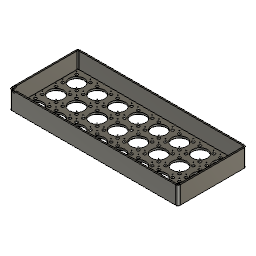
clockclock24 (Autodesk Fusion 360 design; units mm, degrees)
Autodesk Fusion 360 part; units mm, degrees
(part 1 of 2)
sketch "Sketch2" plane through (0, 0, 0) normal (0, 0, 1) x (1, 0, 0)
  circle A0 centre (0, 0) radius 16.1
  circle A1 centre (-15, 15) radius 0.95
  circle A2 centre (15, 15) radius 0.95
  circle A3 centre (-15, -15) radius 0.95
  circle A4 centre (15, -15) radius 0.95
  circle A5 centre (59.5, 15) radius 0.95
  circle A6 centre (59.5, -15) radius 0.95
  circle A7 centre (44.5, 0) radius 16.1
  circle A8 centre (29.5, 15) radius 0.95
  circle A9 centre (29.5, -15) radius 0.95
  circle A10 centre (104, 15) radius 0.95
  circle A11 centre (104, -15) radius 0.95
  circle A12 centre (89, 0) radius 16.1
  circle A13 centre (74, 15) radius 0.95
  circle A14 centre (74, -15) radius 0.95
  circle A15 centre (148.5, 15) radius 0.95
  circle A16 centre (148.5, -15) radius 0.95
  circle A17 centre (133.5, 0) radius 16.1
  circle A18 centre (118.5, 15) radius 0.95
  circle A19 centre (118.5, -15) radius 0.95
  circle A20 centre (193, 15) radius 0.95
  circle A21 centre (193, -15) radius 0.95
  circle A22 centre (178, 0) radius 16.1
  circle A23 centre (163, 15) radius 0.95
  circle A24 centre (163, -15) radius 0.95
  circle A25 centre (237.5, 15) radius 0.95
  circle A26 centre (237.5, -15) radius 0.95
  circle A27 centre (222.5, 0) radius 16.1
  circle A28 centre (207.5, 15) radius 0.95
  circle A29 centre (207.5, -15) radius 0.95
  circle A30 centre (282, 15) radius 0.95
  circle A31 centre (282, -15) radius 0.95
  circle A32 centre (267, 0) radius 16.1
  circle A33 centre (252, 15) radius 0.95
  circle A34 centre (252, -15) radius 0.95
  circle A35 centre (326.5, 15) radius 0.95
  circle A36 centre (326.5, -15) radius 0.95
  circle A37 centre (311.5, 0) radius 16.1
  circle A38 centre (296.5, 15) radius 0.95
  circle A39 centre (296.5, -15) radius 0.95
  circle A40 centre (15, 59.5) radius 0.95
  circle A41 centre (15, 29.5) radius 0.95
  circle A42 centre (0, 44.5) radius 16.1
  circle A43 centre (-15, 59.5) radius 0.95
  circle A44 centre (-15, 29.5) radius 0.95
  circle A45 centre (59.5, 59.5) radius 0.95
  circle A46 centre (59.5, 29.5) radius 0.95
  circle A47 centre (44.5, 44.5) radius 16.1
  circle A48 centre (29.5, 59.5) radius 0.95
  circle A49 centre (29.5, 29.5) radius 0.95
  circle A50 centre (104, 59.5) radius 0.95
  circle A51 centre (104, 29.5) radius 0.95
  circle A52 centre (89, 44.5) radius 16.1
  circle A53 centre (74, 59.5) radius 0.95
  circle A54 centre (74, 29.5) radius 0.95
  circle A55 centre (148.5, 59.5) radius 0.95
  circle A56 centre (148.5, 29.5) radius 0.95
  circle A57 centre (133.5, 44.5) radius 16.1
  circle A58 centre (118.5, 59.5) radius 0.95
  circle A59 centre (118.5, 29.5) radius 0.95
  circle A60 centre (193, 59.5) radius 0.95
  circle A61 centre (193, 29.5) radius 0.95
  circle A62 centre (178, 44.5) radius 16.1
  circle A63 centre (163, 59.5) radius 0.95
  circle A64 centre (163, 29.5) radius 0.95
  circle A65 centre (237.5, 59.5) radius 0.95
  circle A66 centre (237.5, 29.5) radius 0.95
  circle A67 centre (222.5, 44.5) radius 16.1
  circle A68 centre (207.5, 59.5) radius 0.95
  circle A69 centre (207.5, 29.5) radius 0.95
  circle A70 centre (282, 59.5) radius 0.95
  circle A71 centre (282, 29.5) radius 0.95
  circle A72 centre (267, 44.5) radius 16.1
  circle A73 centre (252, 59.5) radius 0.95
  circle A74 centre (252, 29.5) radius 0.95
  circle A75 centre (326.5, 59.5) radius 0.95
  circle A76 centre (326.5, 29.5) radius 0.95
  circle A77 centre (311.5, 44.5) radius 16.1
  circle A78 centre (296.5, 59.5) radius 0.95
  circle A79 centre (296.5, 29.5) radius 0.95
  circle A80 centre (15, 104) radius 0.95
  circle A81 centre (15, 74) radius 0.95
  circle A82 centre (0, 89) radius 16.1
  circle A83 centre (-15, 104) radius 0.95
  circle A84 centre (-15, 74) radius 0.95
  circle A85 centre (59.5, 104) radius 0.95
  circle A86 centre (59.5, 74) radius 0.95
  circle A87 centre (44.5, 89) radius 16.1
  circle A88 centre (29.5, 104) radius 0.95
  circle A89 centre (29.5, 74) radius 0.95
  circle A90 centre (104, 104) radius 0.95
  circle A91 centre (104, 74) radius 0.95
  circle A92 centre (89, 89) radius 16.1
  circle A93 centre (74, 104) radius 0.95
  circle A94 centre (74, 74) radius 0.95
  circle A95 centre (148.5, 104) radius 0.95
  circle A96 centre (148.5, 74) radius 0.95
  circle A97 centre (133.5, 89) radius 16.1
  circle A98 centre (118.5, 104) radius 0.95
  circle A99 centre (118.5, 74) radius 0.95
  circle A100 centre (193, 104) radius 0.95
  circle A101 centre (193, 74) radius 0.95
  circle A102 centre (178, 89) radius 16.1
  circle A103 centre (163, 104) radius 0.95
  circle A104 centre (163, 74) radius 0.95
  circle A105 centre (237.5, 104) radius 0.95
  circle A106 centre (237.5, 74) radius 0.95
  circle A107 centre (222.5, 89) radius 16.1
  circle A108 centre (207.5, 104) radius 0.95
  circle A109 centre (207.5, 74) radius 0.95
  circle A110 centre (282, 104) radius 0.95
  circle A111 centre (282, 74) radius 0.95
  circle A112 centre (267, 89) radius 16.1
  circle A113 centre (252, 104) radius 0.95
  circle A114 centre (252, 74) radius 0.95
  circle A115 centre (326.5, 104) radius 0.95
  circle A116 centre (326.5, 74) radius 0.95
  circle A117 centre (311.5, 89) radius 16.1
  circle A118 centre (296.5, 104) radius 0.95
  circle A119 centre (296.5, 74) radius 0.95
  line L0 (-22, -30) -> (333.5, -30)
  line L1 (338.5, -25) -> (338.5, 114)
  line L2 (333.5, 119) -> (-22, 119)
  line L3 (-27, 114) -> (-27, -25)
  arc A120 (338.5, 114) -> (333.5, 119) centre (333.5, 114) ccw
  arc A121 (-22, 119) -> (-27, 114) centre (-22, 114) ccw
  arc A122 (-27, -25) -> (-22, -30) centre (-22, -25) ccw
  arc A123 (333.5, -30) -> (338.5, -25) centre (333.5, -25) ccw
  point P0 (44.5, 0)
  point P1 (89, 0)
  point P2 (133.5, 0)
  point P3 (178, 0)
  point P4 (222.5, 0)
  point P5 (267, 0)
  point P6 (311.5, 0)
  point P7 (0, 44.5)
  point P8 (44.5, 44.5)
  point P9 (89, 44.5)
  point P10 (133.5, 44.5)
  point P11 (178, 44.5)
  point P12 (222.5, 44.5)
  point P13 (267, 44.5)
  point P14 (311.5, 44.5)
  point P15 (0, 89)
  point P16 (44.5, 89)
  point P17 (89, 89)
  point P18 (133.5, 89)
  point P19 (178, 89)
  point P20 (222.5, 89)
  point P21 (267, 89)
  point P22 (311.5, 89)
  point P23 (-27, -30)
  point P24 (338.5, -30)
  dimension "d3" = 32.2
  dimension "d5" = 15
  dimension "d6" = 15
  dimension "d7" = 1.9
  dimension "d10" = 30
  dimension "d11" = -30
  dimension "d14" = 311.5
  dimension "d15" = 89
  dimension "d17" = 27
  dimension "d18" = 27
  dimension "d19" = 30
  dimension "d20" = 30
  dimension "d22" = 365.5
  dimension "d41" = 5
  constraint coincident A0.centre origin
  constraint horizontal L0
  constraint vertical L1
  constraint horizontal L2
  constraint vertical L3
  constraint tangent L1 A120
  constraint tangent L2 A120
  constraint tangent L2 A121
  constraint tangent L3 A121
  constraint equal A120 A121
  constraint coincident P23 L0
  constraint coincident P23 L3
  constraint tangent L0 A122
  constraint tangent L3 A122
  constraint equal A120 A122
  constraint coincident P24 L0
  constraint coincident P24 L1
  constraint tangent L0 A123
  constraint tangent L1 A123
  constraint equal A120 A123
  measures "d3" diameter of A0
  measures "d5" horizontal distance of A0.centre A1.centre
  measures "d6" vertical distance of A0.centre A1.centre
  measures "d7" diameter of A1
  measures "d17" distance of P7 L3
  measures "d18" distance of P14 L1
  measures "d19" distance of P22 L2
  measures "d20" distance of P6 L0
  measures "d22" distance of P23 P24
  measures "d41" radius of A120
extrude "Extrude2" add sketch "Sketch2" along normal blind 5 contours A1 | A2 | A3 | A4 | A5 | A6 | A8 | A9 | A10 | A11 | A13 | A14 | A15 | A16 | A18 | A19 | A20 | A21 | A23 | A24 | A25 | A26 | A28 | A29 | A30 | A31 | A33 | A34 | A35 | A36 | A38 | A39 | A40 | A41 | A43 | A44 | A45 | A46 | A48 | A49 | A50 | A51 | A53 | A54 | A55 | A56 | A58 | A59 | A60 | A61 | A63 | A64 | A65 | A66 | A68 | A69 | A70 | A71 | A73 | A74 | A75 | A76 | A78 | A79 | A80 | A81 | A83 | A84 | A85 | A86 | A88 | A89 | A90 | A91 | A93 | A94 | A95 | A96 | A98 | A99 | A100 | A101 | A103 | A104 | A105 | A106 | A108 | A109 | A110 | A111 | A113 | A114 | A115 | A116 | A118 | A119 | L0 L1 L2 L3 A120 A121 A122 A123 makes body 1
extrude "Extrude3" add sketch "Sketch2" along normal blind 11 contours A1 | A2 | A3 | A4 | A5 | A6 | A8 | A9 | A10 | A11 | A13 | A14 | A15 | A16 | A18 | A19 | A20 | A21 | A23 | A24 | A25 | A26 | A28 | A29 | A30 | A31 | A33 | A34 | A35 | A36 | A38 | A39 | A40 | A41 | A43 | A44 | A45 | A46 | A48 | A49 | A50 | A51 | A53 | A54 | A55 | A56 | A58 | A59 | A60 | A61 | A63 | A64 | A65 | A66 | A68 | A69 | A70 | A71 | A73 | A74 | A75 | A76 | A78 | A79 | A80 | A81 | A83 | A84 | A85 | A86 | A88 | A89 | A90 | A91 | A93 | A94 | A95 | A96 | A98 | A99 | A100 | A101 | A103 | A104 | A105 | A106 | A108 | A109 | A110 | A111 | A113 | A114 | A115 | A116 | A118 | A119 bodies 1
extrude "Extrude5" add sketch "Sketch2" along normal blind 40 thin wall 3 on the right open curves L3 A122 L0 A123 L1 A120 L2 A121 bodies 1
fillet "Fillet1" radius 2 96 edges at (-15.8857, -14.6565, 5) (14.1143, -14.6565, 5) (28.6143, -14.6565, 5) (58.6143, -14.6565, 5) (58.6143, 15.3435, 5) (28.6143, 15.3435, 5) (14.1143, 15.3435, 5) (-15.8857, 15.3435, 5) (-15.8857, 29.8435, 5) (-15.8857, 59.8435, 5) (-15.8857, 74.3435, 5) (-15.8857, 104.3435, 5) (14.1143, 104.3435, 5) (28.6143, 104.3435, 5) (58.6143, 104.3435, 5) (73.1143, 104.3435, 5) (73.1143, 74.3435, 5) (58.6143, 74.3435, 5) (28.6143, 59.8435, 5) (14.1143, 59.8435, 5) (14.1143, 74.3435, 5) (28.6143, 74.3435, 5) (58.6143, 59.8435, 5) (73.1143, 59.8435, 5) (58.6143, 29.8435, 5) (73.1143, 29.8435, 5) (28.6143, 29.8435, 5) (14.1143, 29.8435, 5) (73.1143, 15.3435, 5) (73.1143, -14.6565, 5) (103.1143, -14.6565, 5) (103.1143, 15.3435, 5) (103.1143, 29.8435, 5) (103.1143, 59.8435, 5) (103.1143, 74.3435, 5) (103.1143, 104.3435, 5) (117.6143, 104.3435, 5) (117.6143, 74.3435, 5) (117.6143, 59.8435, 5) (117.6143, 29.8435, 5) (117.6143, 15.3435, 5) (117.6143, -14.6565, 5) (147.6143, -14.6565, 5) (147.6143, 15.3435, 5) (147.6143, 29.8435, 5) (147.6143, 59.8435, 5) (147.6143, 74.3435, 5) (147.6143, 104.3435, 5) (162.1143, 104.3435, 5) (162.1143, 74.3435, 5) (162.1143, 59.8435, 5) (162.1143, 29.8435, 5) (162.1143, 15.3435, 5) (162.1143, -14.6565, 5) (192.1143, -14.6565, 5) (192.1143, 15.3435, 5) (192.1143, 29.8435, 5) (192.1143, 59.8435, 5) (192.1143, 74.3435, 5) (192.1143, 104.3435, 5) (206.6143, 104.3435, 5) (236.6143, 104.3435, 5) (251.1143, 104.3435, 5) (281.1143, 104.3435, 5) (295.6143, 104.3435, 5) (206.6143, 74.3435, 5) (236.6143, 74.3435, 5) (251.1143, 74.3435, 5) (281.1143, 74.3435, 5) (295.6143, 74.3435, 5) (295.6143, 59.8435, 5) (281.1143, 59.8435, 5) (251.1143, 59.8435, 5) (236.6143, 59.8435, 5) (206.6143, 59.8435, 5) (206.6143, 29.8435, 5) (236.6143, 29.8435, 5) (251.1143, 29.8435, 5) (281.1143, 29.8435, 5) (295.6143, 29.8435, 5) (325.6143, 29.8435, 5) (325.6143, 15.3435, 5) (295.6143, 15.3435, 5) (281.1143, 15.3435, 5) (251.1143, 15.3435, 5) (325.6143, -14.6565, 5) (295.6143, -14.6565, 5) (281.1143, -14.6565, 5) (251.1143, -14.6565, 5) (236.6143, -14.6565, 5) (236.6143, 15.3435, 5) (206.6143, 15.3435, 5) (206.6143, -14.6565, 5) (325.6143, 104.3435, 5) (325.6143, 74.3435, 5) (325.6143, 59.8435, 5) on bodies 1
sketch "DXF_PCB3_2026-08-19_AutoCAD2007" plane through (0, 0, 0) normal (0, 0, 1) x (1, 0, 0)
  line L0 (-17, -130.4333) -> (-17, -0.301)
  arc A0 (-12, -135.4333) -> (-17, -130.4333) centre (-11.9982, -130.4314) cw
  arc A1 (17, -130.4333) -> (12, -135.4333) centre (11.9982, -130.4314) cw
  line L1 (12, -135.4333) -> (-12, -135.4333)
  arc A2 (12, 4.699) -> (17, -0.301) centre (11.9982, -0.3028) cw
  line L2 (17, -0.301) -> (17, -130.4333)
  line L3 (-12, 4.699) -> (12, 4.699)
  arc A3 (-17, -0.301) -> (-12, 4.699) centre (-11.9982, -0.3028) cw
  arc A4 (-11.722, 1) -> (-15.278, 1) centre (-13.5, 1) ccw
  arc A5 (-15.278, 1) -> (-11.722, 1) centre (-13.5, 1) ccw
  arc A6 (11.722, 1) -> (15.278, 1) centre (13.5, 1) ccw
  arc A7 (15.278, 1) -> (11.722, 1) centre (13.5, 1) ccw
  arc A8 (-11.849, -131.0003) -> (-15.405, -131.0003) centre (-13.627, -131.0003) ccw
  arc A9 (-15.405, -131.0003) -> (-11.849, -131.0003) centre (-13.627, -131.0003) ccw
  arc A10 (11.595, -131.0003) -> (15.151, -131.0003) centre (13.373, -131.0003) ccw
  arc A11 (15.151, -131.0003) -> (11.595, -131.0003) centre (13.373, -131.0003) ccw
  arc A12 (0.4999, -121.4122) -> (1.9999, -121.4122) centre (1.2499, -121.4122) ccw
  arc A13 (1.9999, -121.4122) -> (0.4999, -121.4122) centre (1.2499, -121.4122) ccw
  arc A14 (1.9999, -121.4122) -> (0.4999, -121.4122) centre (1.2499, -121.4122) ccw
  arc A15 (0.4999, -121.4122) -> (1.9999, -121.4122) centre (1.2499, -121.4122) ccw
  arc A16 (0.4999, -121.4122) -> (1.9999, -121.4122) centre (1.2499, -121.4122) ccw
  arc A17 (1.9999, -121.4122) -> (0.4999, -121.4122) centre (1.2499, -121.4122) ccw
  arc A18 (-1.9999, -121.4122) -> (-0.4999, -121.4122) centre (-1.2499, -121.4122) ccw
  arc A19 (-0.4999, -121.4122) -> (-1.9999, -121.4122) centre (-1.2499, -121.4122) ccw
  arc A20 (-1.9999, -121.4122) -> (-0.4999, -121.4122) centre (-1.2499, -121.4122) ccw
  arc A21 (-0.4999, -121.4122) -> (-1.9999, -121.4122) centre (-1.2499, -121.4122) ccw
  arc A22 (-1.9999, -121.4122) -> (-0.4999, -121.4122) centre (-1.2499, -121.4122) ccw
  arc A23 (-0.4999, -121.4122) -> (-1.9999, -121.4122) centre (-1.2499, -121.4122) ccw
  arc A24 (0.47, -96.0122) -> (2.07, -96.0122) centre (1.27, -96.0122) ccw
  arc A25 (2.07, -96.0122) -> (0.47, -96.0122) centre (1.27, -96.0122) ccw
  arc A26 (0.47, -96.0122) -> (2.07, -96.0122) centre (1.27, -96.0122) ccw
  arc A27 (2.07, -96.0122) -> (0.47, -96.0122) centre (1.27, -96.0122) ccw
  arc A28 (2.07, -96.0122) -> (0.47, -96.0122) centre (1.27, -96.0122) ccw
  arc A29 (0.47, -96.0122) -> (2.07, -96.0122) centre (1.27, -96.0122) ccw
  arc A30 (-2.07, -96.0122) -> (-0.47, -96.0122) centre (-1.27, -96.0122) ccw
  arc A31 (-0.47, -96.0122) -> (-2.07, -96.0122) centre (-1.27, -96.0122) ccw
  arc A32 (-2.07, -96.0122) -> (-0.47, -96.0122) centre (-1.27, -96.0122) ccw
  arc A33 (-0.47, -96.0122) -> (-2.07, -96.0122) centre (-1.27, -96.0122) ccw
  arc A34 (-2.07, -96.0122) -> (-0.47, -96.0122) centre (-1.27, -96.0122) ccw
  arc A35 (-0.47, -96.0122) -> (-2.07, -96.0122) centre (-1.27, -96.0122) ccw
  line L4 (-7.1, -63.6671) -> (-7.1, -63.6671)
  arc A36 (-7.1, -63.6671) -> (-8.9, -63.6671) centre (-8, -63.6671) ccw
  arc A37 (-8.9, -63.6671) -> (-7.1, -63.6671) centre (-8, -63.6671) ccw
  arc A38 (-8.9, -63.6671) -> (-7.1, -63.6671) centre (-8, -63.6671) ccw
  arc A39 (-7.1, -63.6671) -> (-8.9, -63.6671) centre (-8, -63.6671) ccw
  line L5 (-7.1, -63.6671) -> (-7.1, -63.6671)
  line L6 (-7.1, -63.6671) -> (-7.1, -63.6671)
  arc A40 (-7.1, -63.6671) -> (-8.9, -63.6671) centre (-8, -63.6671) ccw
  arc A41 (-8.9, -63.6671) -> (-7.1, -63.6671) centre (-8, -63.6671) ccw
  arc A42 (-7.1, -66.167) -> (-8.9, -66.167) centre (-8, -66.167) ccw
  arc A43 (-8.9, -66.167) -> (-7.1, -66.167) centre (-8, -66.167) ccw
  arc A44 (-7.1, -66.167) -> (-8.9, -66.167) centre (-8, -66.167) ccw
  arc A45 (-8.9, -66.167) -> (-7.1, -66.167) centre (-8, -66.167) ccw
  arc A46 (-7.1, -66.167) -> (-8.9, -66.167) centre (-8, -66.167) ccw
  arc A47 (-8.9, -66.167) -> (-7.1, -66.167) centre (-8, -66.167) ccw
  arc A48 (-7.1, -68.6671) -> (-8.9, -68.6671) centre (-8, -68.6671) ccw
  arc A49 (-8.9, -68.6671) -> (-7.1, -68.6671) centre (-8, -68.6671) ccw
  line L7 (-7.1, -68.6671) -> (-7.1, -68.6671)
  line L8 (-7.1, -68.6671) -> (-7.1, -68.6671)
  arc A50 (-7.1, -68.6671) -> (-8.9, -68.6671) centre (-8, -68.6671) ccw
  arc A51 (-8.9, -68.6671) -> (-7.1, -68.6671) centre (-8, -68.6671) ccw
  arc A52 (-7.1, -68.6671) -> (-8.9, -68.6671) centre (-8, -68.6671) ccw
  line L9 (-7.1, -68.6671) -> (-7.1, -68.6671)
  arc A53 (-8.9, -68.6671) -> (-7.1, -68.6671) centre (-8, -68.6671) ccw
  arc A54 (8.9, -68.6671) -> (7.1, -68.6671) centre (8, -68.6671) ccw
  arc A55 (7.1, -68.6671) -> (8.9, -68.6671) centre (8, -68.6671) ccw
  arc A56 (7.1, -68.6671) -> (8.9, -68.6671) centre (8, -68.6671) ccw
  arc A57 (8.9, -68.6671) -> (7.1, -68.6671) centre (8, -68.6671) ccw
  arc A58 (8.9, -68.6671) -> (7.1, -68.6671) centre (8, -68.6671) ccw
  arc A59 (7.1, -68.6671) -> (8.9, -68.6671) centre (8, -68.6671) ccw
  arc A60 (8.9, -66.1673) -> (7.1, -66.1673) centre (8, -66.1673) ccw
  arc A61 (7.1, -66.1673) -> (8.9, -66.1673) centre (8, -66.1673) ccw
  arc A62 (7.1, -66.1673) -> (8.9, -66.1673) centre (8, -66.1673) ccw
  arc A63 (8.9, -66.1673) -> (7.1, -66.1673) centre (8, -66.1673) ccw
  arc A64 (8.9, -66.1673) -> (7.1, -66.1673) centre (8, -66.1673) ccw
  arc A65 (7.1, -66.1673) -> (8.9, -66.1673) centre (8, -66.1673) ccw
  arc A66 (7.1, -63.6671) -> (8.9, -63.6671) centre (8, -63.6671) ccw
  arc A67 (8.9, -63.6671) -> (7.1, -63.6671) centre (8, -63.6671) ccw
  arc A68 (7.1, -63.6671) -> (8.9, -63.6671) centre (8, -63.6671) ccw
  arc A69 (8.9, -63.6671) -> (7.1, -63.6671) centre (8, -63.6671) ccw
  arc A70 (7.1, -63.6671) -> (8.9, -63.6671) centre (8, -63.6671) ccw
  arc A71 (8.9, -63.6671) -> (7.1, -63.6671) centre (8, -63.6671) ccw
  arc A72 (7.112, -12.573) -> (8.636, -12.573) centre (7.874, -12.573) ccw
  arc A73 (8.636, -12.573) -> (7.112, -12.573) centre (7.874, -12.573) ccw
  arc A74 (8.636, -12.573) -> (7.112, -12.573) centre (7.874, -12.573) ccw
  arc A75 (7.112, -12.573) -> (8.636, -12.573) centre (7.874, -12.573) ccw
  arc A76 (8.636, -12.573) -> (7.112, -12.573) centre (7.874, -12.573) ccw
  arc A77 (7.112, -12.573) -> (8.636, -12.573) centre (7.874, -12.573) ccw
  arc A78 (4.572, -12.573) -> (6.096, -12.573) centre (5.334, -12.573) ccw
  arc A79 (6.096, -12.573) -> (4.572, -12.573) centre (5.334, -12.573) ccw
  arc A80 (6.096, -12.573) -> (4.572, -12.573) centre (5.334, -12.573) ccw
  arc A81 (4.572, -12.573) -> (6.096, -12.573) centre (5.334, -12.573) ccw
  arc A82 (6.096, -12.573) -> (4.572, -12.573) centre (5.334, -12.573) ccw
  arc A83 (4.572, -12.573) -> (6.096, -12.573) centre (5.334, -12.573) ccw
  arc A84 (2.032, -12.573) -> (3.556, -12.573) centre (2.794, -12.573) ccw
  arc A85 (3.556, -12.573) -> (2.032, -12.573) centre (2.794, -12.573) ccw
  arc A86 (3.556, -12.573) -> (2.032, -12.573) centre (2.794, -12.573) ccw
  arc A87 (2.032, -12.573) -> (3.556, -12.573) centre (2.794, -12.573) ccw
  arc A88 (3.556, -12.573) -> (2.032, -12.573) centre (2.794, -12.573) ccw
  arc A89 (2.032, -12.573) -> (3.556, -12.573) centre (2.794, -12.573) ccw
  arc A90 (-0.508, -12.573) -> (1.016, -12.573) centre (0.254, -12.573) ccw
  arc A91 (1.016, -12.573) -> (-0.508, -12.573) centre (0.254, -12.573) ccw
  arc A92 (1.016, -12.573) -> (-0.508, -12.573) centre (0.254, -12.573) ccw
  arc A93 (-0.508, -12.573) -> (1.016, -12.573) centre (0.254, -12.573) ccw
  arc A94 (1.016, -12.573) -> (-0.508, -12.573) centre (0.254, -12.573) ccw
  arc A95 (-0.508, -12.573) -> (1.016, -12.573) centre (0.254, -12.573) ccw
  arc A96 (-1.524, -12.573) -> (-3.048, -12.573) centre (-2.286, -12.573) ccw
  arc A97 (-3.048, -12.573) -> (-1.524, -12.573) centre (-2.286, -12.573) ccw
  arc A98 (-3.048, -12.573) -> (-1.524, -12.573) centre (-2.286, -12.573) ccw
  arc A99 (-1.524, -12.573) -> (-3.048, -12.573) centre (-2.286, -12.573) ccw
  arc A100 (-3.048, -12.573) -> (-1.524, -12.573) centre (-2.286, -12.573) ccw
  arc A101 (-1.524, -12.573) -> (-3.048, -12.573) centre (-2.286, -12.573) ccw
  arc A102 (-5.588, -12.573) -> (-4.064, -12.573) centre (-4.826, -12.573) ccw
  arc A103 (-4.064, -12.573) -> (-5.588, -12.573) centre (-4.826, -12.573) ccw
  arc A104 (-4.064, -12.573) -> (-5.588, -12.573) centre (-4.826, -12.573) ccw
  arc A105 (-5.588, -12.573) -> (-4.064, -12.573) centre (-4.826, -12.573) ccw
  arc A106 (-4.064, -12.573) -> (-5.588, -12.573) centre (-4.826, -12.573) ccw
  arc A107 (-5.588, -12.573) -> (-4.064, -12.573) centre (-4.826, -12.573) ccw
  arc A108 (-6.604, -12.573) -> (-8.128, -12.573) centre (-7.366, -12.573) ccw
  arc A109 (-8.128, -12.573) -> (-6.604, -12.573) centre (-7.366, -12.573) ccw
  arc A110 (-6.604, -12.573) -> (-8.128, -12.573) centre (-7.366, -12.573) ccw
  arc A111 (-8.128, -12.573) -> (-6.604, -12.573) centre (-7.366, -12.573) ccw
  arc A112 (-6.604, -12.573) -> (-8.128, -12.573) centre (-7.366, -12.573) ccw
  arc A113 (-8.128, -12.573) -> (-6.604, -12.573) centre (-7.366, -12.573) ccw
  arc A114 (-8.128, -27.8131) -> (-6.604, -27.8131) centre (-7.366, -27.8131) ccw
  arc A115 (-6.604, -27.8131) -> (-8.128, -27.8131) centre (-7.366, -27.8131) ccw
  arc A116 (-6.604, -27.8131) -> (-8.128, -27.8131) centre (-7.366, -27.8131) ccw
  arc A117 (-8.128, -27.8131) -> (-6.604, -27.8131) centre (-7.366, -27.8131) ccw
  arc A118 (-6.604, -27.8131) -> (-8.128, -27.8131) centre (-7.366, -27.8131) ccw
  arc A119 (-8.128, -27.8131) -> (-6.604, -27.8131) centre (-7.366, -27.8131) ccw
  arc A120 (-5.588, -27.8131) -> (-4.064, -27.8131) centre (-4.826, -27.8131) ccw
  arc A121 (-4.064, -27.8131) -> (-5.588, -27.8131) centre (-4.826, -27.8131) ccw
  arc A122 (-4.064, -27.8131) -> (-5.588, -27.8131) centre (-4.826, -27.8131) ccw
  arc A123 (-5.588, -27.8131) -> (-4.064, -27.8131) centre (-4.826, -27.8131) ccw
  arc A124 (-5.588, -27.8131) -> (-4.064, -27.8131) centre (-4.826, -27.8131) ccw
  arc A125 (-4.064, -27.8131) -> (-5.588, -27.8131) centre (-4.826, -27.8131) ccw
  arc A126 (-3.048, -27.8131) -> (-1.524, -27.8131) centre (-2.286, -27.8131) ccw
  arc A127 (-1.524, -27.8131) -> (-3.048, -27.8131) centre (-2.286, -27.8131) ccw
  arc A128 (-3.048, -27.8131) -> (-1.524, -27.8131) centre (-2.286, -27.8131) ccw
  arc A129 (-1.524, -27.8131) -> (-3.048, -27.8131) centre (-2.286, -27.8131) ccw
  arc A130 (-3.048, -27.8131) -> (-1.524, -27.8131) centre (-2.286, -27.8131) ccw
  arc A131 (-1.524, -27.8131) -> (-3.048, -27.8131) centre (-2.286, -27.8131) ccw
  arc A132 (-0.508, -27.8131) -> (1.016, -27.8131) centre (0.254, -27.8131) ccw
  arc A133 (1.016, -27.8131) -> (-0.508, -27.8131) centre (0.254, -27.8131) ccw
  arc A134 (-0.508, -27.8131) -> (1.016, -27.8131) centre (0.254, -27.8131) ccw
  arc A135 (1.016, -27.8131) -> (-0.508, -27.8131) centre (0.254, -27.8131) ccw
  arc A136 (1.016, -27.8131) -> (-0.508, -27.8131) centre (0.254, -27.8131) ccw
  arc A137 (-0.508, -27.8131) -> (1.016, -27.8131) centre (0.254, -27.8131) ccw
  arc A138 (2.032, -27.8131) -> (3.556, -27.8131) centre (2.794, -27.8131) ccw
  arc A139 (3.556, -27.8131) -> (2.032, -27.8131) centre (2.794, -27.8131) ccw
  arc A140 (3.556, -27.8131) -> (2.032, -27.8131) centre (2.794, -27.8131) ccw
  arc A141 (2.032, -27.8131) -> (3.556, -27.8131) centre (2.794, -27.8131) ccw
  arc A142 (3.556, -27.8131) -> (2.032, -27.8131) centre (2.794, -27.8131) ccw
  arc A143 (2.032, -27.8131) -> (3.556, -27.8131) centre (2.794, -27.8131) ccw
  arc A144 (4.572, -27.8131) -> (6.096, -27.8131) centre (5.334, -27.8131) ccw
  arc A145 (6.096, -27.8131) -> (4.572, -27.8131) centre (5.334, -27.8131) ccw
  arc A146 (6.096, -27.8131) -> (4.572, -27.8131) centre (5.334, -27.8131) ccw
  arc A147 (4.572, -27.8131) -> (6.096, -27.8131) centre (5.334, -27.8131) ccw
  arc A148 (6.096, -27.8131) -> (4.572, -27.8131) centre (5.334, -27.8131) ccw
  arc A149 (4.572, -27.8131) -> (6.096, -27.8131) centre (5.334, -27.8131) ccw
  arc A150 (7.112, -27.8131) -> (8.636, -27.8131) centre (7.874, -27.8131) ccw
  arc A151 (8.636, -27.8131) -> (7.112, -27.8131) centre (7.874, -27.8131) ccw
  arc A152 (8.636, -27.8131) -> (7.112, -27.8131) centre (7.874, -27.8131) ccw
  arc A153 (7.112, -27.8131) -> (8.636, -27.8131) centre (7.874, -27.8131) ccw
  arc A154 (7.112, -27.8131) -> (8.636, -27.8131) centre (7.874, -27.8131) ccw
  arc A155 (8.636, -27.8131) -> (7.112, -27.8131) centre (7.874, -27.8131) ccw
  arc A156 (-8.0404, -0.0001) -> (-9.7404, -0.0001) centre (-8.8904, -0.0001) ccw
  arc A157 (-9.7404, -0.0001) -> (-8.0404, -0.0001) centre (-8.8904, -0.0001) ccw
  arc A158 (-8.0404, -0.0001) -> (-9.7404, -0.0001) centre (-8.8904, -0.0001) ccw
  arc A159 (-9.7404, -0.0001) -> (-8.0404, -0.0001) centre (-8.8904, -0.0001) ccw
  arc A160 (-8.0404, -0.0001) -> (-9.7404, -0.0001) centre (-8.8904, -0.0001) ccw
  arc A161 (-9.7404, -0.0001) -> (-8.0404, -0.0001) centre (-8.8904, -0.0001) ccw
  arc A162 (-5.5004, -0.0001) -> (-7.2004, -0.0001) centre (-6.3504, -0.0001) ccw
  arc A163 (-7.2004, -0.0001) -> (-5.5004, -0.0001) centre (-6.3504, -0.0001) ccw
  arc A164 (-7.2004, -0.0001) -> (-5.5004, -0.0001) centre (-6.3504, -0.0001) ccw
  arc A165 (-5.5004, -0.0001) -> (-7.2004, -0.0001) centre (-6.3504, -0.0001) ccw
  arc A166 (-5.5004, -0.0001) -> (-7.2004, -0.0001) centre (-6.3504, -0.0001) ccw
  arc A167 (-7.2004, -0.0001) -> (-5.5004, -0.0001) centre (-6.3504, -0.0001) ccw
  arc A168 (-2.9604, -0.0001) -> (-4.6604, -0.0001) centre (-3.8104, -0.0001) ccw
  arc A169 (-4.6604, -0.0001) -> (-2.9604, -0.0001) centre (-3.8104, -0.0001) ccw
  arc A170 (-4.6604, -0.0001) -> (-2.9604, -0.0001) centre (-3.8104, -0.0001) ccw
  arc A171 (-2.9604, -0.0001) -> (-4.6604, -0.0001) centre (-3.8104, -0.0001) ccw
  arc A172 (-4.6604, -0.0001) -> (-2.9604, -0.0001) centre (-3.8104, -0.0001) ccw
  arc A173 (-2.9604, -0.0001) -> (-4.6604, -0.0001) centre (-3.8104, -0.0001) ccw
  arc A174 (-0.4204, -0.0001) -> (-2.1204, -0.0001) centre (-1.2704, -0.0001) ccw
  arc A175 (-2.1204, -0.0001) -> (-0.4204, -0.0001) centre (-1.2704, -0.0001) ccw
  arc A176 (-2.1204, -0.0001) -> (-0.4204, -0.0001) centre (-1.2704, -0.0001) ccw
  arc A177 (-0.4204, -0.0001) -> (-2.1204, -0.0001) centre (-1.2704, -0.0001) ccw
  arc A178 (-0.4204, -0.0001) -> (-2.1204, -0.0001) centre (-1.2704, -0.0001) ccw
  arc A179 (-2.1204, -0.0001) -> (-0.4204, -0.0001) centre (-1.2704, -0.0001) ccw
  arc A180 (0.4196, -0.0001) -> (2.1196, -0.0001) centre (1.2696, -0.0001) ccw
  arc A181 (2.1196, -0.0001) -> (0.4196, -0.0001) centre (1.2696, -0.0001) ccw
  arc A182 (2.1196, -0.0001) -> (0.4196, -0.0001) centre (1.2696, -0.0001) ccw
  arc A183 (0.4196, -0.0001) -> (2.1196, -0.0001) centre (1.2696, -0.0001) ccw
  arc A184 (0.4196, -0.0001) -> (2.1196, -0.0001) centre (1.2696, -0.0001) ccw
  arc A185 (2.1196, -0.0001) -> (0.4196, -0.0001) centre (1.2696, -0.0001) ccw
  arc A186 (2.9596, -0.0001) -> (4.6596, -0.0001) centre (3.8096, -0.0001) ccw
  arc A187 (4.6596, -0.0001) -> (2.9596, -0.0001) centre (3.8096, -0.0001) ccw
  arc A188 (2.9596, -0.0001) -> (4.6596, -0.0001) centre (3.8096, -0.0001) ccw
  arc A189 (4.6596, -0.0001) -> (2.9596, -0.0001) centre (3.8096, -0.0001) ccw
  arc A190 (2.9596, -0.0001) -> (4.6596, -0.0001) centre (3.8096, -0.0001) ccw
  arc A191 (4.6596, -0.0001) -> (2.9596, -0.0001) centre (3.8096, -0.0001) ccw
  arc A192 (5.4996, -0.0001) -> (7.1996, -0.0001) centre (6.3496, -0.0001) ccw
  arc A193 (7.1996, -0.0001) -> (5.4996, -0.0001) centre (6.3496, -0.0001) ccw
  arc A194 (5.4996, -0.0001) -> (7.1996, -0.0001) centre (6.3496, -0.0001) ccw
  arc A195 (7.1996, -0.0001) -> (5.4996, -0.0001) centre (6.3496, -0.0001) ccw
  arc A196 (7.1996, -0.0001) -> (5.4996, -0.0001) centre (6.3496, -0.0001) ccw
  arc A197 (5.4996, -0.0001) -> (7.1996, -0.0001) centre (6.3496, -0.0001) ccw
  line L10 (9.677, -0.8501) -> (8.1022, -0.8501)
  line L11 (9.677, 0.8499) -> (9.677, -0.8501)
  line L12 (8.1022, 0.8499) -> (9.677, 0.8499)
  line L13 (8.1022, -0.8501) -> (8.1022, 0.8499)
  line L14 (8.1022, -0.8501) -> (8.1022, 0.8499)
  line L15 (8.1022, 0.8499) -> (9.677, 0.8499)
  line L16 (9.677, 0.8499) -> (9.677, -0.8501)
  line L17 (9.677, -0.8501) -> (8.1022, -0.8501)
  line L18 (8.1022, -0.8501) -> (8.1022, 0.8499)
  line L19 (8.1022, 0.8499) -> (9.677, 0.8499)
  line L20 (9.677, 0.8499) -> (9.677, -0.8501)
  line L21 (9.677, -0.8501) -> (8.1022, -0.8501)
  line L22 (2.151, -128.5243) -> (2.151, -128.5243)
  arc A198 (0.351, -128.5243) -> (2.151, -128.5243) centre (1.251, -128.5243) ccw
  arc A199 (2.151, -128.5243) -> (0.351, -128.5243) centre (1.251, -128.5243) ccw
  arc A200 (0.351, -128.5243) -> (2.151, -128.5243) centre (1.251, -128.5243) ccw
  line L23 (2.151, -128.5243) -> (2.151, -128.5243)
  arc A201 (2.151, -128.5243) -> (0.351, -128.5243) centre (1.251, -128.5243) ccw
  line L24 (2.151, -128.5243) -> (2.151, -128.5243)
  arc A202 (2.151, -128.5243) -> (0.351, -128.5243) centre (1.251, -128.5243) ccw
  arc A203 (0.351, -128.5243) -> (2.151, -128.5243) centre (1.251, -128.5243) ccw
  arc A204 (-2.151, -128.5243) -> (-0.351, -128.5243) centre (-1.251, -128.5243) ccw
  arc A205 (-0.351, -128.5243) -> (-2.151, -128.5243) centre (-1.251, -128.5243) ccw
  line L25 (-0.351, -128.5243) -> (-0.351, -128.5243)
  arc A206 (-2.151, -128.5243) -> (-0.351, -128.5243) centre (-1.251, -128.5243) ccw
  arc A207 (-0.351, -128.5243) -> (-2.151, -128.5243) centre (-1.251, -128.5243) ccw
  line L26 (-0.351, -128.5243) -> (-0.351, -128.5243)
  arc A208 (-2.151, -128.5243) -> (-0.351, -128.5243) centre (-1.251, -128.5243) ccw
  arc A209 (-0.351, -128.5243) -> (-2.151, -128.5243) centre (-1.251, -128.5243) ccw
  line L27 (-0.351, -128.5243) -> (-0.351, -128.5243)
  arc A210 (-8.382, -102.1082) -> (-10.16, -102.1082) centre (-9.271, -102.1082) ccw
  arc A211 (-10.16, -102.1082) -> (-8.382, -102.1082) centre (-9.271, -102.1082) ccw
  arc A212 (-8.382, -102.1082) -> (-10.16, -102.1082) centre (-9.271, -102.1082) ccw
  arc A213 (-10.16, -102.1082) -> (-8.382, -102.1082) centre (-9.271, -102.1082) ccw
  arc A214 (-8.382, -102.1082) -> (-10.16, -102.1082) centre (-9.271, -102.1082) ccw
  arc A215 (-10.16, -102.1082) -> (-8.382, -102.1082) centre (-9.271, -102.1082) ccw
  arc A216 (-8.382, -104.6482) -> (-10.16, -104.6482) centre (-9.271, -104.6482) ccw
  arc A217 (-10.16, -104.6482) -> (-8.382, -104.6482) centre (-9.271, -104.6482) ccw
  arc A218 (-10.16, -104.6482) -> (-8.382, -104.6482) centre (-9.271, -104.6482) ccw
  arc A219 (-8.382, -104.6482) -> (-10.16, -104.6482) centre (-9.271, -104.6482) ccw
  arc A220 (-8.382, -104.6482) -> (-10.16, -104.6482) centre (-9.271, -104.6482) ccw
  arc A221 (-10.16, -104.6482) -> (-8.382, -104.6482) centre (-9.271, -104.6482) ccw
  arc A222 (-8.382, -112.7762) -> (-10.16, -112.7762) centre (-9.271, -112.7762) ccw
  arc A223 (-10.16, -112.7762) -> (-8.382, -112.7762) centre (-9.271, -112.7762) ccw
  arc A224 (-10.16, -112.7762) -> (-8.382, -112.7762) centre (-9.271, -112.7762) ccw
  arc A225 (-8.382, -112.7762) -> (-10.16, -112.7762) centre (-9.271, -112.7762) ccw
  arc A226 (-10.16, -112.7762) -> (-8.382, -112.7762) centre (-9.271, -112.7762) ccw
  arc A227 (-8.382, -112.7762) -> (-10.16, -112.7762) centre (-9.271, -112.7762) ccw
  arc A228 (-10.16, -115.3162) -> (-8.382, -115.3162) centre (-9.271, -115.3162) ccw
  arc A229 (-8.382, -115.3162) -> (-10.16, -115.3162) centre (-9.271, -115.3162) ccw
  arc A230 (-8.382, -115.3162) -> (-10.16, -115.3162) centre (-9.271, -115.3162) ccw
  arc A231 (-10.16, -115.3162) -> (-8.382, -115.3162) centre (-9.271, -115.3162) ccw
  arc A232 (-10.16, -115.3162) -> (-8.382, -115.3162) centre (-9.271, -115.3162) ccw
  arc A233 (-8.382, -115.3162) -> (-10.16, -115.3162) centre (-9.271, -115.3162) ccw
  arc A234 (10.16, -102.1082) -> (8.382, -102.1082) centre (9.271, -102.1082) ccw
  arc A235 (8.382, -102.1082) -> (10.16, -102.1082) centre (9.271, -102.1082) ccw
  arc A236 (10.16, -102.1082) -> (8.382, -102.1082) centre (9.271, -102.1082) ccw
  arc A237 (8.382, -102.1082) -> (10.16, -102.1082) centre (9.271, -102.1082) ccw
  arc A238 (8.382, -102.1082) -> (10.16, -102.1082) centre (9.271, -102.1082) ccw
  arc A239 (10.16, -102.1082) -> (8.382, -102.1082) centre (9.271, -102.1082) ccw
  arc A240 (8.382, -104.6482) -> (10.16, -104.6482) centre (9.271, -104.6482) ccw
  arc A241 (10.16, -104.6482) -> (8.382, -104.6482) centre (9.271, -104.6482) ccw
  arc A242 (8.382, -104.6482) -> (10.16, -104.6482) centre (9.271, -104.6482) ccw
  arc A243 (10.16, -104.6482) -> (8.382, -104.6482) centre (9.271, -104.6482) ccw
  arc A244 (10.16, -104.6482) -> (8.382, -104.6482) centre (9.271, -104.6482) ccw
  arc A245 (8.382, -104.6482) -> (10.16, -104.6482) centre (9.271, -104.6482) ccw
  arc A246 (10.16, -112.7762) -> (8.382, -112.7762) centre (9.271, -112.7762) ccw
  arc A247 (8.382, -112.7762) -> (10.16, -112.7762) centre (9.271, -112.7762) ccw
  arc A248 (8.382, -112.7762) -> (10.16, -112.7762) centre (9.271, -112.7762) ccw
  arc A249 (10.16, -112.7762) -> (8.382, -112.7762) centre (9.271, -112.7762) ccw
  arc A250 (10.16, -112.7762) -> (8.382, -112.7762) centre (9.271, -112.7762) ccw
  arc A251 (8.382, -112.7762) -> (10.16, -112.7762) centre (9.271, -112.7762) ccw
  arc A252 (8.382, -115.3162) -> (10.16, -115.3162) centre (9.271, -115.3162) ccw
  arc A253 (10.16, -115.3162) -> (8.382, -115.3162) centre (9.271, -115.3162) ccw
  arc A254 (8.382, -115.3162) -> (10.16, -115.3162) centre (9.271, -115.3162) ccw
  arc A255 (10.16, -115.3162) -> (8.382, -115.3162) centre (9.271, -115.3162) ccw
  arc A256 (8.382, -115.3162) -> (10.16, -115.3162) centre (9.271, -115.3162) ccw
  arc A257 (10.16, -115.3162) -> (8.382, -115.3162) centre (9.271, -115.3162) ccw
  arc A258 (-8.0404, -44.4999) -> (-9.7404, -44.4999) centre (-8.8904, -44.4999) ccw
  arc A259 (-9.7404, -44.4999) -> (-8.0404, -44.4999) centre (-8.8904, -44.4999) ccw
  arc A260 (-9.7404, -44.4999) -> (-8.0404, -44.4999) centre (-8.8904, -44.4999) ccw
  arc A261 (-8.0404, -44.4999) -> (-9.7404, -44.4999) centre (-8.8904, -44.4999) ccw
  arc A262 (-9.7404, -44.4999) -> (-8.0404, -44.4999) centre (-8.8904, -44.4999) ccw
  arc A263 (-8.0404, -44.4999) -> (-9.7404, -44.4999) centre (-8.8904, -44.4999) ccw
  arc A264 (-7.2004, -44.4999) -> (-5.5004, -44.4999) centre (-6.3504, -44.4999) ccw
  arc A265 (-5.5004, -44.4999) -> (-7.2004, -44.4999) centre (-6.3504, -44.4999) ccw
  arc A266 (-7.2004, -44.4999) -> (-5.5004, -44.4999) centre (-6.3504, -44.4999) ccw
  arc A267 (-5.5004, -44.4999) -> (-7.2004, -44.4999) centre (-6.3504, -44.4999) ccw
  arc A268 (-5.5004, -44.4999) -> (-7.2004, -44.4999) centre (-6.3504, -44.4999) ccw
  arc A269 (-7.2004, -44.4999) -> (-5.5004, -44.4999) centre (-6.3504, -44.4999) ccw
  arc A270 (-2.9604, -44.4999) -> (-4.6604, -44.4999) centre (-3.8104, -44.4999) ccw
  arc A271 (-4.6604, -44.4999) -> (-2.9604, -44.4999) centre (-3.8104, -44.4999) ccw
  arc A272 (-2.9604, -44.4999) -> (-4.6604, -44.4999) centre (-3.8104, -44.4999) ccw
  arc A273 (-4.6604, -44.4999) -> (-2.9604, -44.4999) centre (-3.8104, -44.4999) ccw
  arc A274 (-4.6604, -44.4999) -> (-2.9604, -44.4999) centre (-3.8104, -44.4999) ccw
  arc A275 (-2.9604, -44.4999) -> (-4.6604, -44.4999) centre (-3.8104, -44.4999) ccw
  arc A276 (-0.4204, -44.4999) -> (-2.1204, -44.4999) centre (-1.2704, -44.4999) ccw
  arc A277 (-2.1204, -44.4999) -> (-0.4204, -44.4999) centre (-1.2704, -44.4999) ccw
  arc A278 (-0.4204, -44.4999) -> (-2.1204, -44.4999) centre (-1.2704, -44.4999) ccw
  arc A279 (-2.1204, -44.4999) -> (-0.4204, -44.4999) centre (-1.2704, -44.4999) ccw
  arc A280 (-0.4204, -44.4999) -> (-2.1204, -44.4999) centre (-1.2704, -44.4999) ccw
  arc A281 (-2.1204, -44.4999) -> (-0.4204, -44.4999) centre (-1.2704, -44.4999) ccw
  arc A282 (2.1196, -44.4999) -> (0.4196, -44.4999) centre (1.2696, -44.4999) ccw
  arc A283 (0.4196, -44.4999) -> (2.1196, -44.4999) centre (1.2696, -44.4999) ccw
  arc A284 (0.4196, -44.4999) -> (2.1196, -44.4999) centre (1.2696, -44.4999) ccw
  arc A285 (2.1196, -44.4999) -> (0.4196, -44.4999) centre (1.2696, -44.4999) ccw
  arc A286 (0.4196, -44.4999) -> (2.1196, -44.4999) centre (1.2696, -44.4999) ccw
  arc A287 (2.1196, -44.4999) -> (0.4196, -44.4999) centre (1.2696, -44.4999) ccw
  arc A288 (2.9596, -44.4999) -> (4.6596, -44.4999) centre (3.8096, -44.4999) ccw
  arc A289 (4.6596, -44.4999) -> (2.9596, -44.4999) centre (3.8096, -44.4999) ccw
  arc A290 (2.9596, -44.4999) -> (4.6596, -44.4999) centre (3.8096, -44.4999) ccw
  arc A291 (4.6596, -44.4999) -> (2.9596, -44.4999) centre (3.8096, -44.4999) ccw
  arc A292 (4.6596, -44.4999) -> (2.9596, -44.4999) centre (3.8096, -44.4999) ccw
  arc A293 (2.9596, -44.4999) -> (4.6596, -44.4999) centre (3.8096, -44.4999) ccw
  arc A294 (7.1996, -44.4999) -> (5.4996, -44.4999) centre (6.3496, -44.4999) ccw
  arc A295 (5.4996, -44.4999) -> (7.1996, -44.4999) centre (6.3496, -44.4999) ccw
  arc A296 (5.4996, -44.4999) -> (7.1996, -44.4999) centre (6.3496, -44.4999) ccw
  arc A297 (7.1996, -44.4999) -> (5.4996, -44.4999) centre (6.3496, -44.4999) ccw
  arc A298 (7.1996, -44.4999) -> (5.4996, -44.4999) centre (6.3496, -44.4999) ccw
  arc A299 (5.4996, -44.4999) -> (7.1996, -44.4999) centre (6.3496, -44.4999) ccw
  line L28 (8.1022, -43.6499) -> (9.677, -43.6499)
  line L29 (8.1022, -45.3499) -> (8.1022, -43.6499)
  line L30 (9.677, -45.3499) -> (8.1022, -45.3499)
  line L31 (9.677, -43.6499) -> (9.677, -45.3499)
  line L32 (8.1022, -43.6499) -> (9.677, -43.6499)
  line L33 (9.677, -43.6499) -> (9.677, -45.3499)
  line L34 (8.1022, -45.3499) -> (8.1022, -43.6499)
  line L35 (9.677, -45.3499) -> (8.1022, -45.3499)
  line L36 (9.677, -45.3499) -> (8.1022, -45.3499)
  line L37 (9.677, -43.6499) -> (9.677, -45.3499)
  line L38 (8.1022, -45.3499) -> (8.1022, -43.6499)
  line L39 (8.1022, -43.6499) -> (9.677, -43.6499)
  arc A300 (-8.0404, -88.9997) -> (-9.7404, -88.9997) centre (-8.8904, -88.9997) ccw
  arc A301 (-9.7404, -88.9997) -> (-8.0404, -88.9997) centre (-8.8904, -88.9997) ccw
  arc A302 (-9.7404, -88.9997) -> (-8.0404, -88.9997) centre (-8.8904, -88.9997) ccw
  arc A303 (-8.0404, -88.9997) -> (-9.7404, -88.9997) centre (-8.8904, -88.9997) ccw
  arc A304 (-8.0404, -88.9997) -> (-9.7404, -88.9997) centre (-8.8904, -88.9997) ccw
  arc A305 (-9.7404, -88.9997) -> (-8.0404, -88.9997) centre (-8.8904, -88.9997) ccw
  arc A306 (-5.5004, -88.9997) -> (-7.2004, -88.9997) centre (-6.3504, -88.9997) ccw
  arc A307 (-7.2004, -88.9997) -> (-5.5004, -88.9997) centre (-6.3504, -88.9997) ccw
  arc A308 (-7.2004, -88.9997) -> (-5.5004, -88.9997) centre (-6.3504, -88.9997) ccw
  arc A309 (-5.5004, -88.9997) -> (-7.2004, -88.9997) centre (-6.3504, -88.9997) ccw
  arc A310 (-5.5004, -88.9997) -> (-7.2004, -88.9997) centre (-6.3504, -88.9997) ccw
  arc A311 (-7.2004, -88.9997) -> (-5.5004, -88.9997) centre (-6.3504, -88.9997) ccw
  arc A312 (-2.9604, -88.9997) -> (-4.6604, -88.9997) centre (-3.8104, -88.9997) ccw
  arc A313 (-4.6604, -88.9997) -> (-2.9604, -88.9997) centre (-3.8104, -88.9997) ccw
  arc A314 (-2.9604, -88.9997) -> (-4.6604, -88.9997) centre (-3.8104, -88.9997) ccw
  arc A315 (-4.6604, -88.9997) -> (-2.9604, -88.9997) centre (-3.8104, -88.9997) ccw
  arc A316 (-4.6604, -88.9997) -> (-2.9604, -88.9997) centre (-3.8104, -88.9997) ccw
  arc A317 (-2.9604, -88.9997) -> (-4.6604, -88.9997) centre (-3.8104, -88.9997) ccw
  arc A318 (-0.4204, -88.9997) -> (-2.1204, -88.9997) centre (-1.2704, -88.9997) ccw
  arc A319 (-2.1204, -88.9997) -> (-0.4204, -88.9997) centre (-1.2704, -88.9997) ccw
  arc A320 (-0.4204, -88.9997) -> (-2.1204, -88.9997) centre (-1.2704, -88.9997) ccw
  arc A321 (-2.1204, -88.9997) -> (-0.4204, -88.9997) centre (-1.2704, -88.9997) ccw
  arc A322 (-2.1204, -88.9997) -> (-0.4204, -88.9997) centre (-1.2704, -88.9997) ccw
  arc A323 (-0.4204, -88.9997) -> (-2.1204, -88.9997) centre (-1.2704, -88.9997) ccw
  arc A324 (0.4196, -88.9997) -> (2.1196, -88.9997) centre (1.2696, -88.9997) ccw
  arc A325 (2.1196, -88.9997) -> (0.4196, -88.9997) centre (1.2696, -88.9997) ccw
  arc A326 (0.4196, -88.9997) -> (2.1196, -88.9997) centre (1.2696, -88.9997) ccw
  arc A327 (2.1196, -88.9997) -> (0.4196, -88.9997) centre (1.2696, -88.9997) ccw
  arc A328 (2.1196, -88.9997) -> (0.4196, -88.9997) centre (1.2696, -88.9997) ccw
  arc A329 (0.4196, -88.9997) -> (2.1196, -88.9997) centre (1.2696, -88.9997) ccw
  arc A330 (4.6596, -88.9997) -> (2.9596, -88.9997) centre (3.8096, -88.9997) ccw
  arc A331 (2.9596, -88.9997) -> (4.6596, -88.9997) centre (3.8096, -88.9997) ccw
  arc A332 (4.6596, -88.9997) -> (2.9596, -88.9997) centre (3.8096, -88.9997) ccw
  arc A333 (2.9596, -88.9997) -> (4.6596, -88.9997) centre (3.8096, -88.9997) ccw
  arc A334 (2.9596, -88.9997) -> (4.6596, -88.9997) centre (3.8096, -88.9997) ccw
  arc A335 (4.6596, -88.9997) -> (2.9596, -88.9997) centre (3.8096, -88.9997) ccw
  arc A336 (7.1996, -88.9997) -> (5.4996, -88.9997) centre (6.3496, -88.9997) ccw
  arc A337 (5.4996, -88.9997) -> (7.1996, -88.9997) centre (6.3496, -88.9997) ccw
  arc A338 (7.1996, -88.9997) -> (5.4996, -88.9997) centre (6.3496, -88.9997) ccw
  arc A339 (5.4996, -88.9997) -> (7.1996, -88.9997) centre (6.3496, -88.9997) ccw
  arc A340 (5.4996, -88.9997) -> (7.1996, -88.9997) centre (6.3496, -88.9997) ccw
  arc A341 (7.1996, -88.9997) -> (5.4996, -88.9997) centre (6.3496, -88.9997) ccw
  line L40 (8.1022, -88.1497) -> (9.677, -88.1497)
  line L41 (8.1022, -89.8497) -> (8.1022, -88.1497)
  line L42 (9.677, -89.8497) -> (8.1022, -89.8497)
  line L43 (9.677, -88.1497) -> (9.677, -89.8497)
  line L44 (8.1022, -88.1497) -> (9.677, -88.1497)
  line L45 (9.677, -88.1497) -> (9.677, -89.8497)
  line L46 (8.1022, -89.8497) -> (8.1022, -88.1497)
  line L47 (9.677, -89.8497) -> (8.1022, -89.8497)
  line L48 (8.1022, -89.8497) -> (8.1022, -88.1497)
  line L49 (9.677, -88.1497) -> (9.677, -89.8497)
  line L50 (8.1022, -88.1497) -> (9.677, -88.1497)
  line L51 (9.677, -89.8497) -> (8.1022, -89.8497)
  arc A342 (-0.623, -73.4262) -> (0.877, -73.4262) centre (0.127, -73.4262) ccw
  arc A343 (0.877, -73.4262) -> (-0.623, -73.4262) centre (0.127, -73.4262) ccw
  arc A344 (-0.623, -73.4262) -> (0.877, -73.4262) centre (0.127, -73.4262) ccw
  arc A345 (0.877, -73.4262) -> (-0.623, -73.4262) centre (0.127, -73.4262) ccw
  arc A346 (0.877, -73.4262) -> (-0.623, -73.4262) centre (0.127, -73.4262) ccw
  arc A347 (-0.623, -73.4262) -> (0.877, -73.4262) centre (0.127, -73.4262) ccw
  arc A348 (0.877, -75.9261) -> (-0.623, -75.9261) centre (0.127, -75.9261) ccw
  arc A349 (-0.623, -75.9261) -> (0.877, -75.9261) centre (0.127, -75.9261) ccw
  arc A350 (-0.623, -75.9261) -> (0.877, -75.9261) centre (0.127, -75.9261) ccw
  arc A351 (0.877, -75.9261) -> (-0.623, -75.9261) centre (0.127, -75.9261) ccw
  arc A352 (-0.623, -75.9261) -> (0.877, -75.9261) centre (0.127, -75.9261) ccw
  arc A353 (0.877, -75.9261) -> (-0.623, -75.9261) centre (0.127, -75.9261) ccw
  arc A354 (6.021, -67.4771) -> (5.411, -67.4771) centre (5.716, -67.4771) ccw
  arc A355 (5.411, -67.4771) -> (6.021, -67.4771) centre (5.716, -67.4771) ccw
  arc A356 (4.21, -72.148) -> (3.6, -72.148) centre (3.905, -72.148) ccw
  arc A357 (3.6, -72.148) -> (4.21, -72.148) centre (3.905, -72.148) ccw
  arc A358 (1.7001, -121.4123) -> (0.8, -121.4123) centre (1.25, -121.4123) ccw
  arc A359 (0.8, -121.4123) -> (1.7001, -121.4123) centre (1.25, -121.4123) ccw
  arc A360 (-1.7, -121.4123) -> (-0.8, -121.4123) centre (-1.25, -121.4123) ccw
  arc A361 (-0.8, -121.4123) -> (-1.7, -121.4123) centre (-1.25, -121.4123) ccw
  arc A362 (1.77, -96.0122) -> (0.77, -96.0122) centre (1.27, -96.0122) ccw
  arc A363 (0.77, -96.0122) -> (1.77, -96.0122) centre (1.27, -96.0122) ccw
  arc A364 (-0.77, -96.0122) -> (-1.77, -96.0122) centre (-1.27, -96.0122) ccw
  arc A365 (-1.77, -96.0122) -> (-0.77, -96.0122) centre (-1.27, -96.0122) ccw
  arc A366 (-7.5, -63.667) -> (-8.5, -63.667) centre (-8, -63.667) ccw
  arc A367 (-8.5, -63.667) -> (-7.5, -63.667) centre (-8, -63.667) ccw
  arc A368 (-7.5, -66.167) -> (-8.5, -66.167) centre (-8, -66.167) ccw
  arc A369 (-8.5, -66.167) -> (-7.5, -66.167) centre (-8, -66.167) ccw
  arc A370 (-7.5, -68.667) -> (-8.5, -68.667) centre (-8, -68.667) ccw
  arc A371 (-8.5, -68.667) -> (-7.5, -68.667) centre (-8, -68.667) ccw
  arc A372 (8.5, -68.6673) -> (7.5, -68.6673) centre (8, -68.6673) ccw
  arc A373 (7.5, -68.6673) -> (8.5, -68.6673) centre (8, -68.6673) ccw
  arc A374 (8.5, -66.1673) -> (7.5, -66.1673) centre (8, -66.1673) ccw
  arc A375 (7.5, -66.1673) -> (8.5, -66.1673) centre (8, -66.1673) ccw
  arc A376 (8.5, -63.6673) -> (7.5, -63.6673) centre (8, -63.6673) ccw
  arc A377 (7.5, -63.6673) -> (8.5, -63.6673) centre (8, -63.6673) ccw
  arc A378 (8.3185, -12.573) -> (7.4295, -12.573) centre (7.874, -12.573) ccw
  arc A379 (7.4295, -12.573) -> (8.3185, -12.573) centre (7.874, -12.573) ccw
  arc A380 (5.7785, -12.573) -> (4.8895, -12.573) centre (5.334, -12.573) ccw
  arc A381 (4.8895, -12.573) -> (5.7785, -12.573) centre (5.334, -12.573) ccw
  arc A382 (3.2385, -12.573) -> (2.3495, -12.573) centre (2.794, -12.573) ccw
  arc A383 (2.3495, -12.573) -> (3.2385, -12.573) centre (2.794, -12.573) ccw
  arc A384 (-0.1905, -12.573) -> (0.6985, -12.573) centre (0.254, -12.573) ccw
  arc A385 (0.6985, -12.573) -> (-0.1905, -12.573) centre (0.254, -12.573) ccw
  arc A386 (-1.8415, -12.573) -> (-2.7305, -12.573) centre (-2.286, -12.573) ccw
  arc A387 (-2.7305, -12.573) -> (-1.8415, -12.573) centre (-2.286, -12.573) ccw
  arc A388 (-4.3815, -12.573) -> (-5.2705, -12.573) centre (-4.826, -12.573) ccw
  arc A389 (-5.2705, -12.573) -> (-4.3815, -12.573) centre (-4.826, -12.573) ccw
  arc A390 (-6.9215, -12.573) -> (-7.8105, -12.573) centre (-7.366, -12.573) ccw
  arc A391 (-7.8105, -12.573) -> (-6.9215, -12.573) centre (-7.366, -12.573) ccw
  arc A392 (-7.8105, -27.8131) -> (-6.9215, -27.8131) centre (-7.366, -27.8131) ccw
  arc A393 (-6.9215, -27.8131) -> (-7.8105, -27.8131) centre (-7.366, -27.8131) ccw
  arc A394 (-4.3815, -27.8131) -> (-5.2705, -27.8131) centre (-4.826, -27.8131) ccw
  arc A395 (-5.2705, -27.8131) -> (-4.3815, -27.8131) centre (-4.826, -27.8131) ccw
  arc A396 (-1.8415, -27.8131) -> (-2.7305, -27.8131) centre (-2.286, -27.8131) ccw
  arc A397 (-2.7305, -27.8131) -> (-1.8415, -27.8131) centre (-2.286, -27.8131) ccw
  arc A398 (0.6985, -27.8131) -> (-0.1905, -27.8131) centre (0.254, -27.8131) ccw
  arc A399 (-0.1905, -27.8131) -> (0.6985, -27.8131) centre (0.254, -27.8131) ccw
  arc A400 (2.3495, -27.8131) -> (3.2385, -27.8131) centre (2.794, -27.8131) ccw
  arc A401 (3.2385, -27.8131) -> (2.3495, -27.8131) centre (2.794, -27.8131) ccw
  arc A402 (4.8895, -27.8131) -> (5.7785, -27.8131) centre (5.334, -27.8131) ccw
  arc A403 (5.7785, -27.8131) -> (4.8895, -27.8131) centre (5.334, -27.8131) ccw
  arc A404 (7.4295, -27.8131) -> (8.3185, -27.8131) centre (7.874, -27.8131) ccw
  arc A405 (8.3185, -27.8131) -> (7.4295, -27.8131) centre (7.874, -27.8131) ccw
  arc A406 (-9.4404, -0.0001) -> (-8.3404, -0.0001) centre (-8.8904, -0.0001) ccw
  arc A407 (-8.3404, -0.0001) -> (-9.4404, -0.0001) centre (-8.8904, -0.0001) ccw
  arc A408 (-6.9004, -0.0001) -> (-5.8004, -0.0001) centre (-6.3504, -0.0001) ccw
  arc A409 (-5.8004, -0.0001) -> (-6.9004, -0.0001) centre (-6.3504, -0.0001) ccw
  arc A410 (-3.2604, -0.0001) -> (-4.3604, -0.0001) centre (-3.8104, -0.0001) ccw
  arc A411 (-4.3604, -0.0001) -> (-3.2604, -0.0001) centre (-3.8104, -0.0001) ccw
  arc A412 (-0.7204, -0.0001) -> (-1.8204, -0.0001) centre (-1.2704, -0.0001) ccw
  arc A413 (-1.8204, -0.0001) -> (-0.7204, -0.0001) centre (-1.2704, -0.0001) ccw
  arc A414 (1.8196, -0.0001) -> (0.7196, -0.0001) centre (1.2696, -0.0001) ccw
  arc A415 (0.7196, -0.0001) -> (1.8196, -0.0001) centre (1.2696, -0.0001) ccw
  arc A416 (3.2596, -0.0001) -> (4.3596, -0.0001) centre (3.8096, -0.0001) ccw
  arc A417 (4.3596, -0.0001) -> (3.2596, -0.0001) centre (3.8096, -0.0001) ccw
  arc A418 (6.8996, -0.0001) -> (5.7996, -0.0001) centre (6.3496, -0.0001) ccw
  arc A419 (5.7996, -0.0001) -> (6.8996, -0.0001) centre (6.3496, -0.0001) ccw
  arc A420 (8.3396, -0.0001) -> (9.4397, -0.0001) centre (8.8896, -0.0001) ccw
  arc A421 (9.4397, -0.0001) -> (8.3396, -0.0001) centre (8.8896, -0.0001) ccw
  arc A422 (0.7009, -128.5243) -> (1.801, -128.5243) centre (1.251, -128.5243) ccw
  arc A423 (1.801, -128.5243) -> (0.7009, -128.5243) centre (1.251, -128.5243) ccw
  arc A424 (-0.7009, -128.5243) -> (-1.801, -128.5243) centre (-1.251, -128.5243) ccw
  arc A425 (-1.801, -128.5243) -> (-0.7009, -128.5243) centre (-1.251, -128.5243) ccw
  arc A426 (-9.7282, -102.1082) -> (-8.8138, -102.1082) centre (-9.271, -102.1082) ccw
  arc A427 (-8.8138, -102.1082) -> (-9.7282, -102.1082) centre (-9.271, -102.1082) ccw
  arc A428 (-9.7282, -104.6482) -> (-8.8138, -104.6482) centre (-9.271, -104.6482) ccw
  arc A429 (-8.8138, -104.6482) -> (-9.7282, -104.6482) centre (-9.271, -104.6482) ccw
  arc A430 (-9.7282, -112.7762) -> (-8.8138, -112.7762) centre (-9.271, -112.7762) ccw
  arc A431 (-8.8138, -112.7762) -> (-9.7282, -112.7762) centre (-9.271, -112.7762) ccw
  arc A432 (-8.8138, -115.3162) -> (-9.7282, -115.3162) centre (-9.271, -115.3162) ccw
  arc A433 (-9.7282, -115.3162) -> (-8.8138, -115.3162) centre (-9.271, -115.3162) ccw
  arc A434 (9.7282, -102.1082) -> (8.8138, -102.1082) centre (9.271, -102.1082) ccw
  arc A435 (8.8138, -102.1082) -> (9.7282, -102.1082) centre (9.271, -102.1082) ccw
  arc A436 (9.7282, -104.6482) -> (8.8138, -104.6482) centre (9.271, -104.6482) ccw
  arc A437 (8.8138, -104.6482) -> (9.7282, -104.6482) centre (9.271, -104.6482) ccw
  arc A438 (9.7282, -112.7762) -> (8.8138, -112.7762) centre (9.271, -112.7762) ccw
  arc A439 (8.8138, -112.7762) -> (9.7282, -112.7762) centre (9.271, -112.7762) ccw
  arc A440 (8.8138, -115.3162) -> (9.7282, -115.3162) centre (9.271, -115.3162) ccw
  arc A441 (9.7282, -115.3162) -> (8.8138, -115.3162) centre (9.271, -115.3162) ccw
  arc A442 (-9.4404, -44.4999) -> (-8.3404, -44.4999) centre (-8.8904, -44.4999) ccw
  arc A443 (-8.3404, -44.4999) -> (-9.4404, -44.4999) centre (-8.8904, -44.4999) ccw
  arc A444 (-6.9004, -44.4999) -> (-5.8004, -44.4999) centre (-6.3504, -44.4999) ccw
  arc A445 (-5.8004, -44.4999) -> (-6.9004, -44.4999) centre (-6.3504, -44.4999) ccw